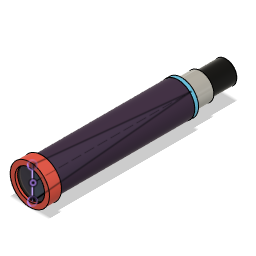
TD Scope CNC v49 (Autodesk Fusion 360 design; units mm, degrees)
part number: Eyepiece
Autodesk Fusion 360 part; units mm, degrees
sketch "Sketch1" plane through (0, 0, 0) normal (0, 0, 1) x (1, 0, 0) in component "Tube"
  circle A0 centre (0, 0) radius 26.85
  circle A1 centre (0, 0) radius 25.55
  dimension "d92" = 51.1
  dimension "d415" = 0
  dimension "d416" = 0
  dimension "d417" = 0
  dimension "d418" = 0
  dimension "d93" = 53.7
  constraint coincident A0.centre A1.centre
  constraint concentric A0 A1
  measures "d92" diameter of A1
  measures "d93" diameter of A0
extrude "Extrude1" add sketch "Sketch1" along normal blind 225.212 makes body 1 in component "Tube"
sketch "Sketch1 (2)" plane through (0, 0, 0) normal (0, 1, 0) x (1, 0, 0) in component "Lens"
  arc A0 (0, -1.845) -> (25, -1.15) centre (0, 448.155) ccw
  line L0 (25, -1.15) -> (25, 0)
  line L1 (25, 0) -> (0, 0) construction
  line L2 (0, -1.845) -> (0, 0) construction
  arc A1 (25, 1.15) -> (0, 1.845) centre (0, -448.155) ccw
  line L3 (25, 1.15) -> (25, 0)
  line L4 (0, -1.845) -> (0, 1.845)
  dimension "d5" = 1.15
  dimension "d7" = 25
  dimension "d9" = 450
  constraint vertical L0
  constraint perpendicular L0 L1
  constraint vertical A0.start L1.end
  constraint coincident L1.end L2.end
  constraint symmetric A0.start L1 A1.end
  constraint symmetric A0.end L1 A1.start
  constraint symmetric A0 L1 A1
  constraint symmetric L0.end L1 L3.end
  constraint vertical A0.centre A0.start
  measures "d5" distance of A0.end L0.end
  measures "d7" horizontal distance of L0.end L1.end
  measures "d9" radius of A0
revolve "Revolve1" add sketch "Sketch1 (2)" angle 360 about axis through (0, 0, 1.845) along (0, 0, -1) separate body makes body 2 in component "Lens"
sketch "Sketch1 (3)" plane through (0, 0, 0) normal (0, 0, 1) x (1, 0, 0) in component "Front Lens Holder"
  circle A0 centre (0, 0) radius 31.104
  circle A1 centre (0, 0) radius 23.4
  dimension "d11" = 62.208
  dimension "d99" = 46.8
  dimension "d46" = 0
  dimension "d47" = 0
  dimension "d48" = 0
  dimension "d49" = 0
  dimension "d380" = 0
  dimension "d381" = 0
  dimension "d382" = 0
  dimension "d383" = 0
  constraint coincident A0.centre A1.centre
  constraint concentric A0 A1
  measures "d11" diameter of A0
  measures "d99" diameter of A1
extrude "Extrude1'" add sketch "Sketch1 (3)" along normal blind 19.05 separate body makes body 3 in component "Front Lens Holder"
sketch "Sketch2" plane through (0, 0, 19.05) normal (0, 0, 1) x (1, 0, 0) in component "Front Lens Holder"
  circle A0 centre (0, 0) radius 23.4
  circle A1 centre (0, 0) radius 31.104
  circle A2 centre (0, 0) radius 27.104
  dimension "d15" = 54.208
  constraint concentric A0 A2
  measures "d15" diameter of A2
extrude "Extrude2" cut sketch "Sketch2" against normal blind 12.75 contours A2 bodies 3 in component "Front Lens Holder"
sketch "Sketch3" plane through (0, 0, 6.3) normal (0, 0, 1) x (1, 0, 0) in component "Front Lens Holder"
  circle A0 centre (0, 0) radius 23.4
  circle A1 centre (0, 0) radius 27.104
  circle A2 centre (0, 0) radius 25.296
  dimension "d18" = 50.592
  constraint coincident A0.centre A1.centre
  measures "d18" diameter of A2
extrude "Extrude3" cut sketch "Sketch3" against normal blind 2.3 contours A2 bodies 3 in component "Front Lens Holder"
sketch "Sketch1 (4)" plane through (0, 0, 0) normal (0, 0, 1) x (1, 0, 0) in component "Front Lens Spacer"
  circle A0 centre (0, 0) radius 26.85
  circle A1 centre (0, 0) radius 23.4
  dimension "d27" = 53.7
  dimension "d28" = 46.8
  dimension "d50" = 0
  dimension "d51" = 0
  dimension "d52" = 0
  dimension "d53" = 0
  dimension "d384" = 0
  dimension "d385" = 0
  dimension "d386" = 0
  dimension "d387" = 0
  constraint coincident A0.centre A1.centre
  constraint concentric A0 A1
  measures "d27" diameter of A0
  measures "d28" diameter of A1
extrude "Extrude1''" add sketch "Sketch1 (4)" along normal blind 3.175 separate body makes body 4 in component "Front Lens Spacer"
sketch "Sketch1 (5)" plane through (0, 0, 0) normal (0, 0, 1) x (1, 0, 0) in component "Rear Mount"
  circle A0 centre (0, 0) radius 26.85
  circle A1 centre (0, 0) radius 21.209
  dimension "d70" = 53.7
  dimension "d71" = 42.418
  dimension "d255" = 0
  dimension "d256" = 0
  dimension "d257" = 0
  dimension "d258" = 0
  constraint coincident A0.centre A1.centre
  measures "d70" diameter of A0
  measures "d71" diameter of A1
extrude "Extrude1'''" add sketch "Sketch1 (5)" along normal blind 6 separate body makes body 5 in component "Rear Mount"
sketch "Sketch3 (2)" plane through (0, 0, 0) normal (0, 0, -1) x (-1, 0, 0) in component "Rear Mount"
  circle A0 centre (0, 0) radius 21.209
  circle A1 centre (0, 0) radius 25.169
  circle A2 centre (0, 0) radius 21.209
  circle A3 centre (0, 0) radius 26.85
  dimension "d406" = 50.338
  constraint concentric A1 A2
  constraint equal A0 A2
  constraint coincident A0.centre A1.centre
  measures "d406" diameter of A1
extrude "Extrude3'" add sketch "Sketch3 (2)" along normal blind 19.05 from surface at -6 contours A1 bodies 5 in component "Rear Mount"
sketch "Sketch1 (6)" plane through (0, 0, -13.05) normal (0, 0, -1) x (-1, 0, 0)
  circle A0 centre (0, 0) radius 25.169
  line L0 (-3, 24.9896) -> (-1.5, 25.05)
  line L1 (-1.5, 25.05) -> (1.5, 25.05)
  line L2 (1.5, 25.05) -> (3, 24.9896)
  line L3 (3, 24.9896) -> (-3, 24.9896)
  line L4 (0, 24.9896) -> (0, 0)
  line L5 (0, 24.9896) -> (0, 25.05) construction
  circle A1 centre (0, 0) radius 21.209
  dimension "d144" = 3
  dimension "d145" = 6
  dimension "d146" = 25.05
  constraint horizontal L1
  constraint midpoint L3 L4.start
  constraint coincident A0.centre L4.end
  constraint horizontal L3
  constraint vertical L4
  constraint coincident A0 L2.end
  constraint equal L0 L2
  constraint midpoint L1 L5.end
  measures "d144" horizontal distance of L0.end L1.end
  measures "d145" horizontal distance of L0.start L2.end
  measures "d146" distance of A0.centre L1
sketch "Sketch1 (7)" plane through (0, 0, 0) normal (0, 0, 1) x (1, 0, 0) in component "Light Stop"
  circle A0 centre (0, 0) radius 23.082
  circle A1 centre (0, 0) radius 6.35
  circle A2 centre (0, 0) radius 10.7226
  circle A3 centre (0, 0) radius 15.7226
  dimension "d331" = 46.164
  dimension "d332" = 12.7
  dimension "d334" = 31.4452
  dimension "d335" = 5
  dimension "d340" = 0
  dimension "d341" = 0
  dimension "d342" = 0
  dimension "d343" = 0
  dimension "d364" = 0
  dimension "d365" = 0
  dimension "d366" = 0
  dimension "d367" = 0
  constraint coincident A0.centre A1.centre
  constraint concentric A0 A1
  constraint concentric A2 A3
  measures "d331" diameter of A0
  measures "d332" diameter of A1
  measures "d334" diameter of A3
  measures "d335" distance of A2 A3
extrude "Extrude1''''" add sketch "Sketch1 (7)" along normal blind 19.05 separate body contours A3 makes body 6 in component "Light Stop"
extrude "Extrude2'" add sketch "Sketch1 (7)" along normal blind 6 bodies 6 in component "Light Stop"
sketch "Sketch1 (8)" plane through (0, 0, 0) normal (0, 0, 1) x (1, 0, 0) in component "Eyepiece Tube"
  circle A0 centre (0, 0) radius 21.082
  circle A1 centre (0, 0) radius 16.2306
  dimension "d396" = 32.4612
  dimension "d397" = 42.164
  constraint coincident A0.centre A1.centre
  constraint concentric A0 A1
  measures "d396" diameter of A1
  measures "d397" diameter of A0
extrude "Extrude1'''''" add sketch "Sketch1 (8)" along normal blind 60 separate body makes body 7 in component "Eyepiece Tube"
sketch "Sketch2 (2)" plane through (0, 0, 0) normal (1, 0, 0) x (0, 0, -1) in component "Eyepiece Tube"
  circle A0 centre (-52.5, 0) radius 1.4
  line L0 (-52.5, 0) -> (0, 0) construction
  line L1 (-60, 21.082) -> (-60, -21.082)
  dimension "d401" = 7.5
  dimension "d402" = 2.8
  constraint coincident A0.centre L0.start
  constraint coincident L0.end origin
  constraint horizontal L0
  measures "d401" distance of A0.centre L1
  measures "d402" diameter of A0
extrude "Extrude2''" cut sketch "Sketch2 (2)" against normal through all bodies 7 in component "Eyepiece Tube"
extrude "Extrude3''" cut 1 faces at (9.2015, -0.8482, 6) along direction (0, 0, -1) up to surface (3.5 mm away) on bodies 6 bodies 6 in component "Light Stop"
sketch "Sketch2 (3)" plane through (0, 0, 0) normal (1, 0, 0) x (0, 0, -1) in component "Lens"
  line L0 (-1.15, 25) -> (-1.15, -25)
  line L1 (0, 0) -> (0, 25)
  line L2 (0, 25) -> (250, 0)
  line L3 (250, 0) -> (0, -25)
  line L4 (0, -25) -> (0, 0)
  line L5 (0, 0) -> (250, 0) construction
  line L6 (0, -23.4) -> (0, 23.4)
  dimension "d91" = 250
  dimension "d155" = 50
  dimension "d560" = 46.8
  constraint coincident L1.start L4.end
  constraint parallel L0 L1
  constraint parallel L1 L4
  constraint equal L1 L4
  constraint horizontal L5
  constraint parallel L0 L6
  constraint midpoint L1.start L6
  measures "d91" horizontal distance of L1.start L2.end
  measures "d155" distance of L1.end L3.end
  measures "d560" distance of L6.start L6.end
sketch "Sketch1 (9)" plane through (0, 0, 0) normal (1, 0, 0) x (0, 0, -1) in component "Eyepiece"
  line L0 (0, 12.45) -> (0, 14.875)
  line L1 (0, 14.875) -> (-16.51, 14.875)
  line L2 (-16.51, 14.875) -> (-16.51, 15.875)
  line L3 (-16.51, 15.875) -> (6.35, 15.875)
  line L4 (6.35, 15.875) -> (6.35, 17.78)
  line L5 (6.35, 17.78) -> (46.99, 17.78)
  line L6 (46.99, 17.78) -> (46.99, 12.5)
  line L7 (46.99, 12.5) -> (44.99, 12.5)
  line L8 (44.99, 12.5) -> (44.99, 0)
  line L9 (44.99, 0) -> (6.35, 0)
  line L10 (6.35, 0) -> (6.35, 14.875)
  line L11 (6.35, 14.875) -> (1, 14.875)
  line L12 (1, 14.875) -> (1, 12.45)
  line L13 (1, 12.45) -> (0, 12.45)
  dimension "d532" = 15.875
  dimension "d533" = 1
  dimension "d534" = 12.45
  dimension "d535" = 14.875
  dimension "d536" = 5.35
  dimension "d537" = 16.51
  dimension "d538" = 17.78
  dimension "d539" = 40.64
  dimension "d540" = 12.5
  dimension "d541" = 2
  constraint perpendicular L1 L2
  constraint perpendicular L2 L3
  constraint perpendicular L3 L4
  constraint perpendicular L4 L5
  constraint perpendicular L5 L6
  constraint perpendicular L6 L7
  constraint perpendicular L7 L8
  constraint perpendicular L9 L10
  constraint perpendicular L11 L12
  constraint horizontal L13
  constraint collinear L1 L11
  constraint horizontal L9
  constraint coincident origin L9
  constraint collinear L4 L10
  constraint coincident origin L0
  constraint vertical L0
  measures "d532" distance of origin L3
  measures "d533" distance of L0.start L12.end
  measures "d534" distance of origin L13
  measures "d535" distance of L9.end L10.end
  measures "d536" distance of L10.end L11.end
  measures "d537" distance of L0.end L1.end
  measures "d538" distance of L5 L9
  measures "d539" distance of L4.end L5.end
  measures "d540" distance of L7.end L8.end
  measures "d541" distance of L6.end L7.end
revolve "Revolve1'" add sketch "Sketch1 (9)" angle 360 about axis through (0, 0, 1.75) along (0, 0, 1) separate body makes body 8 in component "Eyepiece"
fillet "Fillet1" radius 1 2 edges at (-16.5768, 6.4295, -46.99) (-11.6541, 4.5202, -46.99) on bodies 8 in component "Eyepiece"
component "Tube" placed x (1, 0, 0) y (0, 1, 0) z (0, 0, 1) at (0, 0, 0)
component "Lens" placed x (1, 0, 0) y (0, 1, 0) z (0, 0, 1) at (0, 0, 229.537)
component "Front Lens Holder" placed x (1, 0, 0) y (0, -1, 0) z (0, 0, -1) at (0, 0, 234.687)
component "Front Lens Spacer" placed x (1, 0, 0) y (0, 1, 0) z (0, 0, 1) at (0, 0, 225.212)
component "Rear Mount" placed x (1, 0, 0) y (0, -1, 0) z (0, 0, -1) at (0, 0, 0)
component "Light Stop" placed x (1, 0, 0) y (0, -1, 0) z (0, 0, -1) at (0, 0, 30)
component "Eyepiece Tube" placed x (1, 0, 0) y (0, -1, 0) z (0, 0, -1) at (0, 0, 24)
component "Eyepiece" placed x (1, 0, 0) y (0, 1, 0) z (0, 0, 1) at (0, 0, -29.65)
equation "d92 = tubeID"
equation "d95 = tubeLength"
equation "d5 = lensEdgeThickness / 2"
equation "d7 = lensDiameter / 2"
equation "d11 = tubeOD + 2 * ( glueGap + holderExteriorWallThickness )"
equation "d99 = opticalClearance"
equation "d13 = holderStock_p75"
equation "d15 = tubeOD + 2 * glueGap"
equation "d16 = lensEdgeThickness + frontHolderFrontLipThickness - holderStock_p75"
equation "d18 = tubeID - 2 * glueGap"
equation "d19 = -lensEdgeThickness"
equation "d27 = tubeOD"
equation "d28 = opticalClearance"
equation "d29 = lensSpacerThickness"
equation "d70 = tubeOD"
equation "d71 = eyepieceHolderOD + eyepieceHolderSlideGap * 2"
equation "d72 = rearMountLip"
equation "d79 = holderStock_p75"
equation "d146 = ( 50.1 / 2 ) * 1 mm"
equation "d331 = eyepieceHolderOD + 4 mm"
equation "d332 = lightStopDiam"
equation "d334 = eyepieceHolderID - ( glueGap * 4 )"
equation "d335 = lightStopWallThickness"
equation "d336 = holderStock_p75"
equation "d338 = lightStopJointThickness"
equation "d396 = eyepieceHolderID"
equation "d397 = eyepieceHolderOD"
equation "d398 = eyepieceHolderLength"
equation "d406 = tubeID - 3 * glueGap"
equation "d527 = -lightStopWebbingThickness"
equation "d91 = focalLength"
equation "d155 = lensDiameter"
equation "d532 = 1.25 in / 2"
equation "d93 = tubeOD"
equation "lensDiameter = 50 mm"
equation "d560 = opticalClearance"
equation "focalLength = 250 mm"
equation "opticalClearance = 46.8 mm"
equation "tubeID = 51.1 mm"
equation "tubeOD = 53.7 mm"
equation "tubeLength = 225.212 mm"
equation "holderExteriorWallThickness = 4 mm"
equation "glueGap = 0.01 in"
equation "lensSpacerThickness = 0.125 in"
equation "eyepieceHolderOD = 1.66 in"
equation "holderStock_p75 = 0.75 in"
equation "rearMountLip = 6 mm"
equation "eyepieceHolderID = 1.278 in"
equation "holderStock_p5 = 0.5 in"
equation "lightStopDiam = 12.7 mm"
equation "lightStopWallThickness = 5 mm"
equation "lightStopWebbingThickness = 2.5 mm"
equation "lightStopJointThickness = 6 mm"
equation "eyepieceHolderLength = 60 mm"
equation "eyepieceHolderSlideGap = 0.005 in"
equation "frontHolderFrontLipThickness = 4 mm"
equation "lensEdgeThickness = 2.3 mm"
